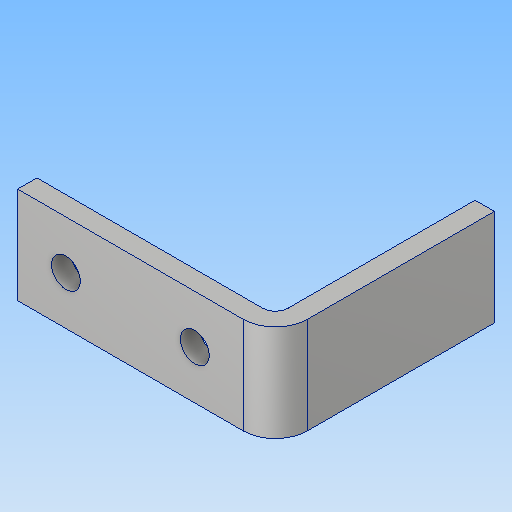
# Autodesk Inventor part: Pancake_Floor Bracket
Saved by Autodesk Inventor 2018.1 (Build 221171000, 171)
## iProperties
Created: 2019-02-12
Part Number: Pancake_Floor Bracket
Material: Aluminum 6061
Document SubType Name: Modeling
Designer: James
Density: 2.7 g/cm^3
Appearance: Aluminum - Flat
Mass: 8.18633 g
Surface Area: 26.1313 cm^2
Volume: 3.03197 cm^3
Author: James
Autodesk Inventor part; units mm, degrees
ref_plane "YZ Plane" through (0, 0, 0) normal (1, 0, 0) x (0, 1, 0)
ref_plane "XZ Plane" through (0, 0, 0) normal (0, 1, 0) x (-1, 0, 0)
ref_plane "XY Plane" through (0, 0, 0) normal (0, 0, 1) x (1, 0, 0)
sketch "Sketch1" plane through (0, 0, 0) normal (0, 1, 0) x (-1, 0, 0)
  line L0 (0, 0) -> (40, 0)
  line L1 (40, 0) -> (40, -3)
  line L2 (40, -3) -> (0, -3)
  line L3 (0, -3) -> (0, 0)
  line L4 (0, 0) -> (3, 0)
  line L5 (3, 0) -> (3, -34)
  line L6 (3, -34) -> (0, -34)
  line L7 (0, -34) -> (0, 0)
  dimension "d0" = 3
  dimension "d1" = 3
  dimension "d2" = 40
  dimension "d3" = 34
  constraints: 16 end point, 4 parallel, 2 horizontal, 2 perpendicular
  measures "d0" distance of L5.end L6.end
  measures "d1" distance of L0.end L1.end
  measures "d2" distance of L0.start L0.end
  measures "d3" distance of L6.end L0.start
extrude "Extrusion1" add sketch "Sketch1" along normal blind 15
fillet "Fillet1" radius 2 1 edges at (-3, 7.5, -3)
fillet "Fillet2" radius 5 1 edges at (0, 7.5, 0)
sketch "Sketch3" plane through (-40, 0, -3) normal (0, 0, -1) x (-1, 0, 0)
  line L0 (-35, 15) -> (0, 15) projected
  line L1 (-35, 0) -> (0, 0) projected
  line L2 (0, 0) -> (0, 15) projected
  line L3 (-40, 0) -> (-40, 15) projected
  line L4 (-40, 0) -> (-40, 15) projected
  point P0 (-7.5, 7.5)
  point P1 (-27.5, 7.5)
  dimension "d20" = 7.5
  dimension "d29" = 7.5
  dimension "d33" = 12.5
  constraints: 1 horizontal alignment
  measures "d20" distance from line of L1 point (-7.5, 7.5)
  measures "d29" distance from line of L2 point (-7.5, 7.5)
  measures "d33" distance from line of point (-27.5, 7.5) L4
hole "Hole2" at (-32.5, 7.5, -3) at (-12.5, 7.5, -3) direction (0, 0, 1) diameter 4.5 end through all clearance for "Socket Head Cap Screw" size "M4" standard "Ansi Metric M Profile"
equation "\"d1\" = d0"
equation "\"d20\" = d19"
equation "\"d19\" = 7.5"
body "Solid1"
